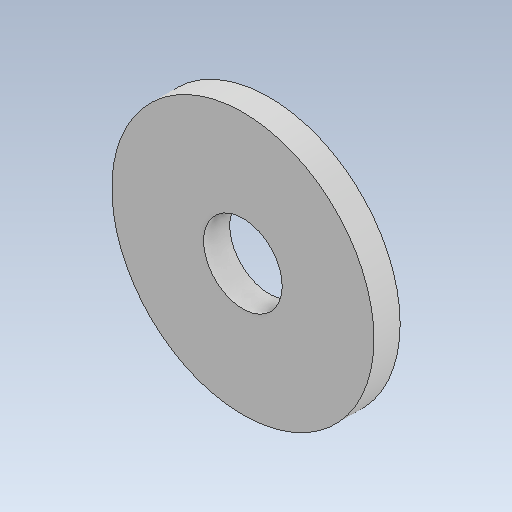
# Autodesk Inventor part: center_holder_retainer
Saved by Autodesk Inventor 2020 (Build 240168000, 168)
## iProperties
Created: 2019-05-02
Part Number: center_holder_retainer
Material: Generic
Document SubType Name: Modeling
Designer: erwin
Density: 1 g/cm^3
Appearance: Default
Author: erwin
Autodesk Inventor part; units mm, degrees
ref_plane "YZ Plane" through (0, 0, 0) normal (1, 0, 0) x (0, 1, 0)
ref_plane "XZ Plane" through (0, 0, 0) normal (0, 1, 0) x (-1, 0, 0)
ref_plane "XY Plane" through (0, 0, 0) normal (0, 0, 1) x (1, 0, 0)
sketch "Sketch1" plane through (0, 0, 0) normal (0, 0, 1) x (1, 0, 0)
  circle A0 centre (4.545, 0) radius 1.5 projected
  circle A1 centre (4.545, 0) radius 3.5 projected
  circle A2 centre (4.545, 0) radius 5
  point P0 (0, 0)
  dimension "d0" = 1.5
  constraints: 1 centre point
  measures "d0" radial gap between concentric circles of A1 A2
extrude "Extrusion1" add sketch "Sketch1" along normal blind 1 contours A1 | A2
body "Solid1"
